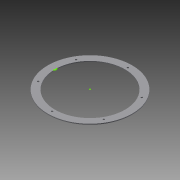
# Autodesk Inventor part: Top Plate
Saved by Autodesk Inventor 2015 (Build 190159000, 159)
## iProperties
Created: 2016-04-12
Part Number: Top Plate
Material: Generic
Document SubType Name: Modeling
Designer: rubenjm
Density: 1 g/cm^3
Appearance: Default
Author: rubenjm
Autodesk Inventor part; units mm, degrees
ref_plane "YZ Plane" through (0, 0, 0) normal (1, 0, 0) x (0, 1, 0)
ref_plane "XZ Plane" through (0, 0, 0) normal (0, 1, 0) x (-1, 0, 0)
ref_plane "XY Plane" through (0, 0, 0) normal (0, 0, 1) x (1, 0, 0)
sketch "Sketch1" plane through (0, 0, 0) normal (0, 1, 0) x (-1, 0, 0)
  circle A0 centre (0, 0) radius 152.4
  dimension "d0" = 304.8
  constraints: 1 centre point, 1 coincident
  measures "d0" diameter of A0
extrude "Extrusion1" add sketch "Sketch1" along normal blind 3.175
sketch "Sketch2" plane through (0, 3.175, 0) normal (0, 1, 0) x (1, 0, 0)
  circle A0 centre (0, 0) radius 137.541 construction
  circle A1 centre (0, -137.541) radius 3.175
  circle A2 centre (119.114, -68.7705) radius 3.175
  circle A3 centre (119.114, 68.7705) radius 3.175
  circle A4 centre (0, 137.541) radius 3.175
  circle A5 centre (-119.114, 68.7705) radius 3.175
  circle A6 centre (-119.114, -68.7705) radius 3.175
  dimension "d3" = 275.082
  dimension "d4" = 6.35
  dimension "d7" = 360
  constraints: 6 centre point, 1 coincident, 1 vertical alignment, 15 other
  measures "d4" diameter of A1
extrude "Extrusion2" cut sketch "Sketch2" against normal through all
sketch "Sketch3" plane through (0, 3.175, 0) normal (0, 1, 0) x (1, 0, 0)
  circle A0 centre (0, 0) radius 127
  dimension "d11" = 254
  constraints: 1 centre point, 1 coincident
  measures "d11" diameter of A0
extrude "Extrusion3" cut sketch "Sketch3" against normal through all
sketch "Sketch4" plane through (0, 3.175, 0) normal (0, 1, 0) x (1, 0, 0)
  line L0 (-123.825, 0) -> (-123.825, 0.7091)
  arc A0 (-123.825, 0.7091) -> (-125.7512, 1.1906) centre (-126.233, -4.8297) ccw
  line L1 (-125.7512, 1.1906) -> (-126.9944, 1.1906)
  arc A1 (-126.9944, 1.1906) -> (-127, 0) centre (0, 0) ccw
  line L2 (-123.825, 0) -> (-123.825, -0.7091)
  arc A2 (-125.7512, -1.1906) -> (-123.825, -0.7091) centre (-126.233, 4.8297) ccw
  line L3 (-125.7512, -1.1906) -> (-126.9944, -1.1906)
  arc A3 (-127, 0) -> (-126.9944, -1.1906) centre (0, 0) ccw
  dimension "d28" = 360
  constraints: 8 end point, 8 point on circle, 4 centre point
body "Solid1"
